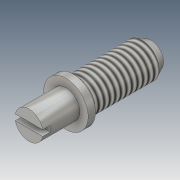
# Autodesk Inventor part: Parafuso da Ponte
Saved by Autodesk Inventor 2016 (Build 200138000, 138)
## iProperties
Created: 2018-12-01
Part Number: Parafuso da Ponte
Material: Aluminum 6061
Document SubType Name: Modeling
Designer: Pedro Mendonça
Density: 2.7 g/cm^3
Appearance: Polished - Small Pyramid Knurl
Author: Pedro Mendonça
Autodesk Inventor part; units mm, degrees
ref_plane "YZ Plane" through (0, 0, 0) normal (1, 0, 0) x (0, 1, 0)
ref_plane "XZ Plane" through (0, 0, 0) normal (0, 1, 0) x (-1, 0, 0)
ref_plane "XY Plane" through (0, 0, 0) normal (0, 0, 1) x (1, 0, 0)
sketch "Sketch1" plane through (0, 0, 0) normal (1, 0, 0) x (0, 1, 0)
  circle A0 centre (0, 0) radius 3.85
  dimension "d0" = 7.7
  constraints: 1 centre point, 1 coincident
  measures "d0" diameter of A0
extrude "Extrusion1" add sketch "Sketch1" along normal blind 16.5
chamfer "Chamfer1" distance 2 distance2 1 1 edges at (0, -3.85, 0) measured on face at (0.5, -3.85, 0)
thread "Thread1" size "M8x1.25" class "6g" standard "ANSI Metric M Profile" full length
sketch "Sketch2" plane through (16.5, 0, 0) normal (1, 0, 0) x (0, 0, -1)
  circle A0 centre (0, 0) radius 3.85 projected
extrude "Extrusion2" add sketch "Sketch2" along normal blind 1 separate body
sketch "Sketch3" plane through (17.5, 0, 0) normal (1, 0, 0) x (0, 0, -1)
  circle A0 centre (0, 0) radius 5
  dimension "d10" = 10
  constraints: 1 centre point, 1 coincident
  measures "d10" diameter of A0
extrude "Extrusion3" add sketch "Sketch3" along normal blind 1.64 bodies 2
sketch "Sketch4" plane through (19.14, 0, 0) normal (1, 0, 0) x (0, 0, -1)
  circle A0 centre (0, 0) radius 3.15
  dimension "d13" = 6.3
  constraints: 1 centre point, 1 coincident
  measures "d13" diameter of A0
extrude "Extrusion4" add sketch "Sketch4" along normal blind 8.3 bodies 2
sketch "Sketch5" plane through (0, 0, 0) normal (0, 1, 0) x (-1, 0, 0)
  line L0 (-29.14, 0.65) -> (-25.74, 0.65)
  line L1 (-25.74, 0.65) -> (-25.74, -0.65)
  line L2 (-25.74, -0.65) -> (-29.14, -0.65)
  line L3 (-29.14, -0.65) -> (-29.14, 0.65)
  line L4 (-27.44, 3.15) -> (-27.44, -3.15) projected
  line L5 (-29.14, 0.65) -> (-25.74, -0.65) construction
  line L6 (-25.74, 0.65) -> (-29.14, -0.65) construction
  point P0 (0, 0)
  point P1 (-27.44, 0)
  dimension "d16" = 3.4
  dimension "d17" = 1.3
  constraints: 12 end point, 3 midpoint, 2 parallel, 1 horizontal, 1 perpendicular
  measures "d16" distance of L1.end L2.end
  measures "d17" distance of L0.end L1.end
extrude "Extrusion5" cut sketch "Sketch5" along normal through all both and the other way through all bodies 2
body "Solid1"
body "Solid2"
